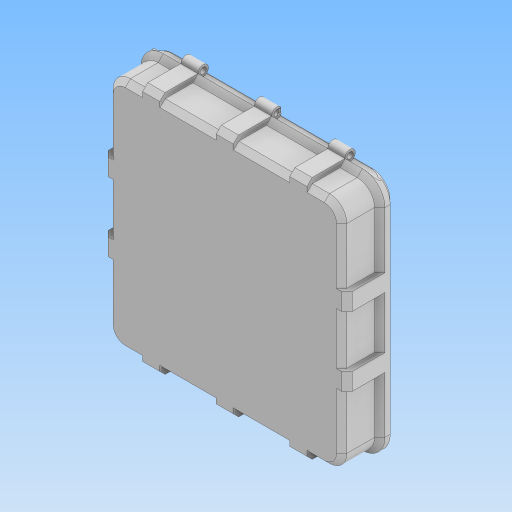
# Autodesk Inventor part: SUMEC_box_top
Saved by Autodesk Inventor 2024 (Build 280153000, 153)
## iProperties
Created: 2023-05-06
Part Number: SUMEC_box_top
Material: Všeobecné
Document SubType Name: Modeling
Designer: Simak
Density: 1 g/cm^3
Appearance: Výchozí
Author: Simak
Autodesk Inventor part; units mm, degrees
ref_plane "YZ Plane" through (0, 0, 0) normal (1, 0, 0) x (0, 1, 0)
ref_plane "XZ Plane" through (0, 0, 0) normal (0, 1, 0) x (-1, 0, 0)
ref_plane "XY Plane" through (0, 0, 0) normal (0, 0, 1) x (1, 0, 0)
sketch "Náčrt1" plane through (0, 0, 0) normal (0, 0, 1) x (1, 0, 0)
  line L0 (0, 0) -> (67.5, 0)
  line L1 (0, 135) -> (0, 0)
  line L2 (67.5, 92.5) -> (70.5, 92.5)
  line L3 (70.5, 92.5) -> (70.5, 82.5)
  line L4 (70.5, 82.5) -> (67.5, 82.5)
  line L5 (67.5, 82.5) -> (67.5, 92.5)
  line L6 (67.5, 52.5) -> (70.5, 52.5)
  line L7 (70.5, 52.5) -> (70.5, 42.5)
  line L8 (70.5, 42.5) -> (67.5, 42.5)
  line L9 (67.5, 42.5) -> (67.5, 52.5)
  line L10 (67.5, 135) -> (67.5, 92.5)
  line L11 (67.5, 42.5) -> (67.5, 0)
  line L12 (67.5, 82.5) -> (67.5, 52.5)
  line L13 (47.5, 135) -> (37.5, 135)
  line L14 (37.5, 135) -> (37.5, 138)
  line L15 (37.5, 138) -> (47.5, 138)
  line L16 (47.5, 138) -> (47.5, 135)
  line L17 (47.5, 135) -> (67.5, 135)
  line L18 (0, 135) -> (5, 135)
  line L19 (5, 135) -> (5, 138)
  line L20 (5, 138) -> (0, 138)
  line L21 (0, 138) -> (0, 135)
  line L22 (5, 135) -> (37.5, 135)
  line L23 (37.5, 0) -> (47.5, 0)
  line L24 (47.5, 0) -> (47.5, -3)
  line L25 (47.5, -3) -> (37.5, -3)
  line L26 (37.5, -3) -> (37.5, 0)
  line L27 (0, 0) -> (5, 0)
  line L28 (5, 0) -> (5, -3)
  line L29 (5, -3) -> (0, -3)
  line L30 (0, -3) -> (0, 0)
  point P0 (47.5, 0)
  dimension "d0" = 135
  dimension "d2" = 3
  dimension "d3" = 10
  dimension "d4" = 30
  dimension "d5" = 20
  dimension "d6" = 5
  dimension "d8" = 67.5
  dimension "d10" = 3
  dimension "d11" = 10
  dimension "d12" = 20
  dimension "d13" = 5
  dimension "d14" = 3
  constraints: 62 end point, 19 equal length, 9 horizontal, 6 perpendicular, 3 vertical, 1 point on line
  measures "d0" distance of L0.end L10.start
  measures "d2" distance of L2.start L2.end
  measures "d3" distance of L2.end L3.end
  measures "d4" distance of L4.end L6.start
  measures "d5" distance of L13.start L10.start
  measures "d6" distance of L19.end L20.end
  measures "d8" horizontal distance of L10.start L20.end
  measures "d10" distance of L23.end L24.end
  measures "d11" distance of L24.end L25.end
  measures "d12" horizontal distance of L0.end L24.end
  measures "d13" distance of L28.end L29.end
  measures "d14" distance of L27.end L28.end
extrude "Vysunutí1" add sketch "Náčrt1" against normal blind 25
sketch "Náčrt2" plane through (0, 0, -25) normal (0, 0, -1) x (-1, 0, 0)
  line L0 (0, -3) -> (0, 138) projected
  line L1 (0, 3) -> (-64.5, 3)
  line L2 (-64.5, 3) -> (-64.5, 132)
  line L3 (-64.5, 132) -> (0, 132)
  line L4 (0, 132) -> (0, 3)
  line L5 (-37.5, 0) -> (-5, 0) projected
  line L6 (-67.5, 42.5) -> (-67.5, 0) projected
  line L7 (-5, 135) -> (-37.5, 135) projected
  point P0 (0, 0)
  point P1 (0, 132)
  dimension "d17" = 3
  dimension "d18" = 3
  dimension "d19" = 3
  constraints: 8 end point, 2 parallel, 1 horizontal, 1 perpendicular, 1 point on line
  measures "d17" distance between parallel lines of L1 L5
  measures "d18" distance between parallel lines of L6 L2
  measures "d19" distance between parallel lines of L7 L3
extrude "Vysunutí2" cut sketch "Náčrt2" against normal blind 22
fillet "Zaoblení1" radius 7 2 edges at (64.5, 3, -14) (64.5, 132, -14)
fillet "Zaoblení2" radius 10 2 edges at (67.5, 0, -12.5) (67.5, 135, -12.5)
chamfer "Zkosení2" distance 3 angle 45 15 edges at (67.5, 67.5, 0) (70.5, 87.5, 0) (67.5, 108.75, 0) (64.5711, 132.0711, 0) (52.5, 135, 0) (42.5, 138, 0) (21.25, 135, 0) (2.5, 138, 0) (70.5, 47.5, 0) (64.5711, 2.9289, 0) (52.5, 0, 0) (67.5, 26.25, 0) (42.5, -3, 0) (21.25, 0, 0) (2.5, -3, 0)
sketch "Náčrt3" plane through (0, 0, -25) normal (0, 0, -1) x (-1, 0, 0)
  line L0 (0, 135) -> (0, 0) projected
  line L1 (-5, -3) -> (0, -3) projected
  line L2 (0, 0) -> (0, -3)
  line L3 (0, -3) -> (-70.5, -3)
  line L4 (-70.5, -3) -> (-70.5, 138)
  line L5 (0, 132) -> (0, 138) projected
  line L6 (-70.5, 138) -> (0, 138)
  line L7 (0, 138) -> (0, -3)
  line L8 (-67.5, 125) -> (-67.5, 92.5) projected
  line L9 (-37.5, 0) -> (-5, 0) projected
  line L10 (-5, 0) -> (0, 0) projected
  line L11 (-47.5, 0) -> (-37.5, 0) projected
  line L12 (-57.5, 0) -> (-47.5, 0) projected
  arc A0 (-67.5, 10) -> (-57.5, 0) centre (-57.5, 10) ccw projected
  line L13 (-67.5, 42.5) -> (-67.5, 10) projected
  line L14 (-67.5, 52.5) -> (-67.5, 42.5) projected
  line L15 (-67.5, 82.5) -> (-67.5, 52.5) projected
  line L16 (-67.5, 92.5) -> (-67.5, 82.5) projected
  arc A1 (-57.5, 135) -> (-67.5, 125) centre (-57.5, 125) ccw projected
  line L17 (-47.5, 135) -> (-57.5, 135) projected
  line L18 (-37.5, 135) -> (-47.5, 135) projected
  line L19 (-5, 135) -> (-37.5, 135) projected
  line L20 (0, 135) -> (-5, 135) projected
  dimension "d32" = 3
  constraints: 10 end point, 3 perpendicular, 1 vertical
  measures "d32" distance between parallel lines of L4 L15
extrude "Vysunutí3" add sketch "Náčrt3" against normal blind 6 contours L20 L19 L18 L17 A1 L8 L16 L15 L14 L13 A0 L12 L11 L9 L10 L2 L1 L3 L4 L6 L5
fillet "Zaoblení3" radius 13 2 edges at (70.5, -3, -22) (70.5, 138, -22)
chamfer "Zkosení3" distance 3 angle 45 9 edges at (70.5, 67.5, -19) (66.6924, 134.1924, -19) (70.5, 108.75, -19) (52.5, 138, -19) (21.25, 138, -19) (66.6924, 0.8076, -19) (52.5, -3, -19) (70.5, 26.25, -19) (21.25, -3, -19)
ref_plane "Pracovní rovina1" through (0, 0, -16) normal (0, 0, -1) x (-1, 0, 0)
sketch "Náčrt12" plane through (0, 0, -16) normal (0, 0, -1) x (-1, 0, 0)
  line L0 (-11.65, 0) -> (-30.85, 0)
  line L1 (-30.85, 0) -> (-30.85, -6)
  line L2 (-30.85, -6) -> (-11.65, -6)
  line L3 (-11.65, -6) -> (-11.65, 0)
  line L4 (-11.65, 0) -> (-5, 0) construction
  line L5 (-37.5, -3) -> (-37.5, 0) construction
  line L6 (-30.85, 0) -> (-37.5, 0) construction
  point P0 (0, 0)
  dimension "d90" = 19.2
  dimension "d91" = 6
  constraints: 12 end point, 2 horizontal, 2 parallel, 2 perpendicular, 1 collinear, 1 horizontal alignment
  measures "d90" distance of L1.end L2.end
  measures "d91" distance of L0.end L1.end
extrude "Vysunutí7" add sketch "Náčrt12" along normal blind 20
chamfer "Zkosení5" distance 6 angle 45 1 edges at (21.25, -6, -16)
sketch "Náčrt14" plane through (30.85, -6, -36) normal (1, 0, 0) x (0, 0, -1)
  line L0 (-11, 6) -> (0, 6) projected
  line L1 (-11, 3) -> (0, 3)
  line L2 (0, 3) -> (0, 6)
  line L3 (0, 6) -> (-11, 6)
  line L4 (-11, 6) -> (-11, 3)
  point P0 (-36, 6)
  constraints: 8 end point, 2 parallel, 1 horizontal, 1 perpendicular
extrude "Vysunutí8" cut sketch "Náčrt14" against normal blind 20
sketch "Náčrt15" plane through (30.85, -6, -22) normal (1, 0, 0) x (0, 0, -1)
  line L0 (14, 3) -> (3, 3) projected
  circle A0 centre (8.5, 3) radius 2
  line L1 (3, 16) -> (3, 3) projected
  point P0 (-22, 6)
  point P1 (6.5, 3)
  point P2 (10.5, 3)
  dimension "d101" = 4
  dimension "d102" = 5.5
  constraints: 1 centre point, 1 midpoint
  measures "d101" diameter of A0
  measures "d102" distance from line of L1 A0.centre
extrude "Vysunutí9" add sketch "Náčrt15" against normal up to surface (19.2 mm away) contours L0 A0 picked at (8.8787, 3.5487)
chamfer "Zkosení6" distance 1 angle 45 10 edges at (30.85, -6, -28.9999) (30.85, -0.0001, -16) (30.85, -3.0001, -18.9999) (11.65, -0.0001, -16) (11.65, -3.0001, -18.9999) (11.65, -6, -28.9999) (21.25, -6, -36) (30.85, -1, -30.5) (11.65, -1, -30.5) (21.25, -3, -36)
sketch "Náčrt16" plane through (30.85, -3, -22) normal (1, 0, 0) x (0, 0, -1)
  arc A0 (5.441, 2.54) -> (5.441, 3.46) centre (5.245, 3) ccw
  line L0 (5.441, 3.46) -> (3, 4.5)
  line L1 (5.441, 2.54) -> (3, 1.5)
  line L2 (3, 1.5) -> (3, 4.5)
  line L3 (3, 4.5) -> (3, 6) construction
  line L4 (3, 1.5) -> (3, 0) construction
  dimension "d108" = 3
  dimension "d109" = 1
  dimension "d110" = 2.7
  constraints: 10 end point, 2 equal length, 2 point on circle, 2 tangent, 1 centre point, 1 vertical, 1 vertical alignment
  measures "d108" distance of L1.end L0.end
  measures "d109" diameter of A0
  measures "d110" distance of L0.end A0.centre
sketch "Náčrt17" plane through (0, 0, -25) normal (0, 0, -1) x (-1, 0, 0)
  line L0 (0, 0) -> (-57.5, 0)
  arc A0 (-67.5, 10) -> (-57.5, 0) centre (-57.5, 10) ccw projected
  arc A1 (-57.5, 135) -> (-67.5, 125) centre (-57.5, 125) ccw projected
  line L1 (-67.5, 10) -> (-67.5, 125)
  line L2 (-57.5, 135) -> (0, 135)
  constraints: 6 end point, 4 tangent, 1 horizontal
sweep "Tažení3" add profiles "Náčrt16" path "Náčrt17" path curves L0 A0 L1 A1 L2
sketch "Náčrt18" plane through (47.5, 132, 0) normal (1, 0, 0) x (0, 0, -1)
  circle A0 centre (25, 6) radius 3
  point P0 (0, -132)
  dimension "d115" = 6
  constraints: 1 centre point
  measures "d115" diameter of A0
extrude "Vysunutí10" cut sketch "Náčrt18" against normal through all
sketch "Náčrt19" plane through (37.5, 138, -3) normal (0, 1, 0) x (1, 0, 0)
  line L0 (9.85, 19) -> (9.85, 22)
  line L1 (0, 19) -> (9.85, 19)
  line L2 (9.85, 22) -> (0, 22)
  line L3 (0, 19) -> (0, 22)
  line L4 (-32.5, 19) -> (-32.5, 20.375)
  arc A0 (-34.125, 22) -> (-32.5, 20.375) centre (-32.5, 22) ccw
  line L5 (-34.125, 22) -> (-37.5, 22)
  line L6 (-37.5, 22) -> (-37.5, 19)
  line L7 (-32.5, 19) -> (-37.5, 19)
  line L8 (20, 22) -> (20, 19) projected
  point P0 (-37.5, -3)
  dimension "d126" = 10.15
  dimension "d188" = 1.625
  dimension "d189" = 3
  constraints: 16 end point, 4 horizontal, 4 vertical, 2 point on circle, 1 centre point, 1 horizontal alignment, 1 point on line
  measures "d126" distance from line of L8 L0.end
  measures "d188" radius of A0
  measures "d189" distance between parallel lines of L2 L1
revolve "Rotace3" add sketch "Náčrt19" angle 360 about axis through (47.35, 138, -25) along (-1, 0, 0)
ref_plane "Pracovní rovina2" through (42.425, 138, -28) normal (0, 0, -1) x (-1, 0, 0)
sketch "Náčrt20" plane through (42.425, 138, -28) normal (0, 0, -1) x (-1, 0, 0)
  arc A0 (37.425, -1.625) -> (37.425, 1.625) centre (37.425, 0) ccw projected
  line L0 (37.425, 1.625) -> (38.025, 1.1)
  line L1 (38.025, 1.1) -> (38.025, -1.1)
  line L2 (38.025, -1.1) -> (37.425, -1.625)
  line L3 (37.425, -1.625) -> (37.425, 1.625) projected
  line L4 (37.425, 1.625) -> (37.425, -1.625)
  point P0 (42.425, -138)
  dimension "d186" = 48.814
  dimension "d187" = 0.6
  constraints: 8 end point, 1 equal length, 1 point on circle, 1 vertical
  measures "d186" angle of L3 L2
  measures "d187" distance between parallel lines of L3 L1
extrude "Vysunutí11" cut sketch "Náčrt20" against normal blind 3 contours L3 L0 L1 L2
fillet "Zaoblení4" radius 0.5 2 edges at (4.4, 136.9, -26.9129) (4.4, 139.1, -26.9129)
sketch "Náčrt22" plane through (47.5, 132, 0) normal (-1, 0, 0) x (0, 0, 1)
  line L0 (-25, 6) -> (-22, 6) projected
  line L1 (-25, 4.5) -> (-25, 6) projected
  arc A0 (-26.9097, 3.6863) -> (-22, 6) centre (-25, 6) ccw projected
  line L2 (-26.9097, 3.6863) -> (-25, 4.5) projected
  point P0 (0, -132)
extrude "Vysunutí13" add sketch "Náčrt22" along normal up to next
sketch "Náčrt27" plane through (47.35, 138, -22) normal (1, 0, 0) x (0, 0, -1)
  arc A0 (4.9097, -2.3137) -> (0, 0) centre (3, 0) ccw projected
  point P0 (-22, -138)
  point P1 (3, 0)
  constraints: 1 coincident
hole "Díra1" at (47.35, 138, -25) direction (1, 0, 0) diameter 6 end through all
sketch "Náčrt28" plane through (47.35, 138, -25) normal (1, 0, 0) x (0, -0.4262804, -0.9045911)
  arc A0 (2.7138, -1.2788) -> (-2.7138, -1.2788) centre (0, 0) ccw projected
  point P0 (36.2119, -135.4906)
  point P1 (0, 0)
  constraints: 1 coincident
hole "Díra2" at (47.35, 138, -25) direction (-1, 0, 0) diameter 3.5 depth 9.85
mirror "Zrcadlit2" about plane through (0, -3, 0) normal (-1, 0, 0)
